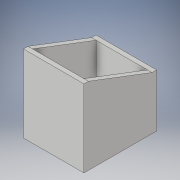
# Autodesk Inventor part: gingerRackHolder
Saved by Autodesk Inventor 2019 (Build 230136000, 136)
## iProperties
Created: 2018-06-30
Part Number: gingerRackHolder
Material: Generic
Document SubType Name: Modeling
Designer: SnoBotics
Density: 1 g/cm^3
Appearance: Default
Author: SnoBotics
Autodesk Inventor part; units mm, degrees
ref_plane "YZ Plane" through (0, 0, 0) normal (1, 0, 0) x (0, 1, 0)
ref_plane "XZ Plane" through (0, 0, 0) normal (0, 1, 0) x (-1, 0, 0)
ref_plane "XY Plane" through (0, 0, 0) normal (0, 0, 1) x (1, 0, 0)
sketch "Sketch1" plane through (0, 0, 0) normal (0, 1, 0) x (-1, 0, 0)
  line L0 (31.75, 38.1) -> (-31.75, 38.1)
  line L1 (-31.75, 38.1) -> (-31.75, -38.1)
  line L2 (-31.75, -38.1) -> (31.75, -38.1)
  line L3 (31.75, -38.1) -> (31.75, 38.1)
  line L4 (31.75, 38.1) -> (-31.75, -38.1) construction
  line L5 (-31.75, 38.1) -> (31.75, -38.1) construction
  point P0 (0, 0)
  dimension "d0" = 63.5
  dimension "d1" = 76.2
  constraints: 12 end point, 2 midpoint, 2 parallel, 1 horizontal, 1 perpendicular
  measures "d0" distance of L0.start L0.end
  measures "d1" distance of L2.end L0.start
extrude "Extrusion1" add sketch "Sketch1" against normal blind 4.7625
sketch "Sketch2" plane through (0, 0, 0) normal (0, 1, 0) x (1, 0, 0)
  line L0 (-31.75, -38.1) -> (-31.75, 38.1) projected
  line L1 (31.75, 38.1) -> (31.75, -38.1) projected
  line L2 (-31.75, 38.1) -> (31.75, 38.1)
  line L3 (31.75, 38.1) -> (31.75, 33.3375)
  line L4 (31.75, 33.3375) -> (-31.75, 33.3375)
  line L5 (-31.75, 33.3375) -> (-31.75, 38.1)
  point P0 (0, 0)
  dimension "d4" = 4.7625
  constraints: 8 end point, 2 parallel, 1 horizontal, 1 perpendicular, 1 point on line
  measures "d4" distance between parallel lines of L2 L4
extrude "Extrusion2" add sketch "Sketch2" along normal blind 50.8
sketch "Sketch3" plane through (0, 0, 0) normal (0, 1, 0) x (1, 0, 0)
  line L0 (31.75, 38.1) -> (31.75, -38.1) projected
  line L1 (-31.75, -38.1) -> (31.75, -38.1)
  line L2 (31.75, -38.1) -> (31.75, -33.3375)
  line L3 (31.75, -33.3375) -> (-31.75, -33.3375)
  line L4 (-31.75, -33.3375) -> (-31.75, -38.1)
  point P0 (0, 0)
  dimension "d7" = 4.7625
  constraints: 8 end point, 2 parallel, 1 horizontal, 1 perpendicular, 1 point on line
  measures "d7" distance between parallel lines of L3 L1
extrude "Extrusion3" add sketch "Sketch3" along normal blind 76.2
sketch "Sketch4" plane through (31.75, -4.7625, 38.1) normal (1, 0, 0) x (0, 0, -1)
  line L0 (4.7625, 4.7625) -> (4.7625, 80.9625) projected
  line L1 (71.4375, 4.7625) -> (71.4375, 55.5625) projected
  line L2 (4.7625, 80.9625) -> (71.4375, 55.5625)
  line L3 (71.4375, 55.5625) -> (71.4375, 4.7625)
  line L4 (71.4375, 4.7625) -> (4.7625, 4.7625) projected
  line L5 (71.4375, 4.7625) -> (4.7625, 4.7625)
  line L6 (4.7625, 4.7625) -> (4.7625, 80.9625)
  point P0 (38.1, 4.7625)
  constraints: 8 end point, 2 perpendicular, 1 collinear
extrude "Extrusion4" add sketch "Sketch4" against normal blind 4.7625
sketch "Sketch5" plane through (-31.75, -4.7625, -38.1) normal (-1, 0, 0) x (0, 0, 1)
  line L0 (71.4375, 80.9625) -> (4.7625, 55.5625) projected
  line L1 (4.7625, 55.5625) -> (71.4375, 80.9625)
  line L2 (4.7625, 4.7625) -> (71.4375, 4.7625) projected
  line L3 (71.4375, 80.9625) -> (71.4375, 4.7625)
  line L4 (71.4375, 4.7625) -> (4.7625, 4.7625)
  line L5 (4.7625, 4.7625) -> (4.7625, 55.5625) projected
  line L6 (4.7625, 4.7625) -> (4.7625, 55.5625)
  point P0 (38.1, 4.7625)
  constraints: 8 end point, 3 perpendicular, 1 collinear
extrude "Extrusion5" add sketch "Sketch5" against normal blind 4.7625
equation "\"d0\" = width"
equation "\"d1\" = depth"
equation "\"d2\" = wallThickness"
equation "\"d4\" = wallThickness"
equation "\"d5\" = rearHeight"
equation "\"d7\" = wallThickness"
equation "\"d8\" = frontHeight"
equation "\"d10\" = wallThickness"
equation "\"d12\" = wallThickness"
equation "\"depth\" = 76.2"
equation "\"width\" = 63.5"
equation "\"frontHeight\" = 76.2"
equation "\"rearHeight\" = 50.8"
equation "\"wallThickness\" = 4.7625"
body "Solid1"
